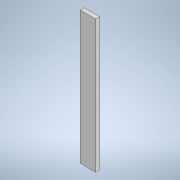
# Autodesk Inventor part: Ruler_1
Saved by Autodesk Inventor 2020 (Build 240168000, 168)
## iProperties
Created: 2021-02-07
Part Number: Ruler_1
Material: Generic
Document SubType Name: Modeling
Designer: moham
Density: 1 g/cm^3
Appearance: Default
Author: moham
Autodesk Inventor part; units mm, degrees
ref_plane "YZ Plane" through (0, 0, 0) normal (1, 0, 0) x (0, 1, 0)
ref_plane "XZ Plane" through (0, 0, 0) normal (0, 1, 0) x (-1, 0, 0)
ref_plane "XY Plane" through (0, 0, 0) normal (0, 0, 1) x (1, 0, 0)
sketch "Sketch1" plane through (0, 0, 0) normal (0, 0, 1) x (1, 0, 0)
  line L0 (-2, -17) -> (2, -17)
  line L1 (2, -17) -> (2, 17)
  line L2 (2, 17) -> (-2, 17)
  line L3 (-2, 17) -> (-2, -17)
  line L4 (-2, -17) -> (2, 17) construction
  line L5 (2, -17) -> (-2, 17) construction
  point P0 (0, 0)
  constraints: 12 end point, 2 midpoint, 2 parallel, 1 horizontal, 1 perpendicular
extrude "Extrusion1" add sketch "Sketch1" along normal blind 1
body "Solid1"
